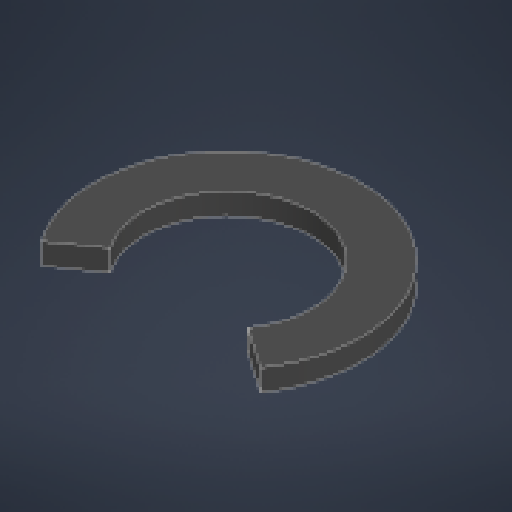
# Autodesk Inventor part: c_ring
Saved by Autodesk Inventor 2026.1 (Build 301233020, 233B)
## iProperties
Created: 2025-12-16
Part Number: c_ring
Material: 고무, 검은색
Document SubType Name: Modeling
Designer: jaewook
Density: 0.93 g/cm^3
Appearance: 고무 - 검은색
Author: jaewook
Autodesk Inventor part; units mm, degrees
ref_plane "YZ Plane" through (0, 0, 0) normal (1, 0, 0) x (0, 1, 0)
ref_plane "XZ Plane" through (0, 0, 0) normal (0, 1, 0) x (-1, 0, 0)
ref_plane "XY Plane" through (0, 0, 0) normal (0, 0, 1) x (1, 0, 0)
sketch "스케치1" plane through (0, 0, 0) normal (1, 0, 0) x (0, 1, 0)
  line L0 (-1.3, -10.2) -> (1.3, -10.2)
  line L1 (1.3, -10.2) -> (1.3, -16.2)
  line L2 (1.3, -16.2) -> (-1.3, -16.2)
  line L3 (-1.3, -16.2) -> (-1.3, -10.2)
  line L4 (-1.3, -10.2) -> (1.3, -16.2) construction
  line L5 (1.3, -10.2) -> (-1.3, -16.2) construction
  line L6 (-2.1884, 0) -> (2.1884, 0)
  point P0 (0, 0)
  point P1 (0, -13.2)
  point P2 (0, 0)
  dimension "d0" = 2.6
  dimension "d1" = 6
  dimension "d2" = 10.2
  constraints: 14 end point, 3 midpoint, 2 horizontal, 2 parallel, 1 coincident, 1 perpendicular, 1 vertical alignment
  measures "d0" distance of L1.end L2.end
  measures "d1" distance of L0.end L1.end
  measures "d2" distance from line of L0 point (0, 0)
revolve "회전1" add sketch "스케치1" angle 250 mid plane about axis through (0, -2.1884, 0) along (0, 1, 0)
